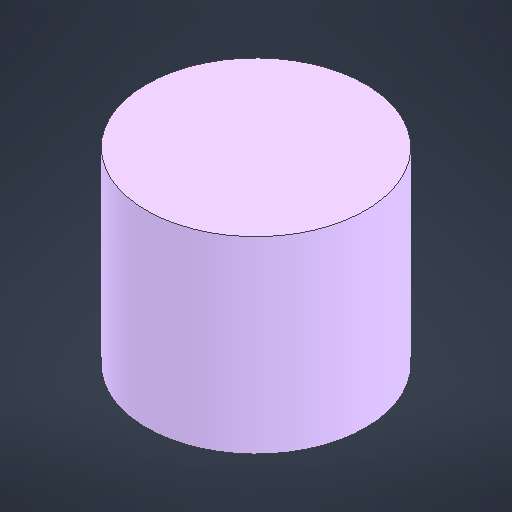
# Autodesk Inventor part: RotaryEncoderKnob
Saved by Autodesk Inventor 2026.2 (Build 302298000, 298)
## iProperties
Created: 2026-02-15
Part Number: RotaryEncoderKnob
Material: Generic
Document SubType Name: Modeling
Designer: bh
Density: 1 g/cm^3
Appearance: Default
Author: bh
Autodesk Inventor part; units mm, degrees
ref_plane "YZ Plane" through (0, 0, 0) normal (1, 0, 0) x (0, 1, 0)
ref_plane "XZ Plane" through (0, 0, 0) normal (0, 1, 0) x (-1, 0, 0)
ref_plane "XY Plane" through (0, 0, 0) normal (0, 0, 1) x (1, 0, 0)
sketch "Sketch2" plane through (0, 0, 0) normal (0, 1, 0) x (-1, 0, 0)
  circle A0 centre (0, 0) radius 10
  dimension "d0" = 20
  constraints: 1 centre point, 1 coincident
  measures "d0" diameter of A0
extrude "Extrusion1" add sketch "Sketch2" along normal blind 20
sketch "Sketch3" plane through (0, 0, 0) normal (0, -1, 0) x (1, 0, 0)
  circle A0 centre (0, 0) radius 4.15
  dimension "d3" = 8.3
  constraints: 1 centre point, 1 coincident
  measures "d3" diameter of A0
extrude "Extrusion2" cut sketch "Sketch3" against normal blind 12.4
sketch "Sketch4" plane through (0, 12.4, 0) normal (0, -1, 0) x (1, 0, 0)
  circle A0 centre (0, 0) radius 4.15 projected
  circle A1 centre (0, 0) radius 3.2
  line L0 (3.2, 0) -> (-1.7, 0)
  line L1 (-1.7, 0) -> (-1.7, -3.7858)
  line L2 (-1.7, 0) -> (-1.7, 3.7858)
  point P0 (-1.7, 2.7111)
  point P1 (-1.7, -2.7111)
  dimension "d16" = 6.4
  dimension "d17" = 4.9
  constraints: 6 end point, 2 point on circle, 1 coincident, 1 horizontal, 1 point on line, 1 vertical, 3 other
  measures "d17" distance of L0.start L0.end
extrude "Extrusion3" cut sketch "Sketch4" against normal blind 6.7 contours A1 L0 L2 | L1 L0 A1
sketch "Sketch8" plane through (0, 0, 0) normal (0, -1, 0) x (1, 0, 0)
  circle A0 centre (0, 0) radius 9.1
  dimension "d18" = 18.2
  constraints: 1 centre point, 1 coincident
  measures "d18" diameter of A0
extrude "Extrusion7" cut sketch "Sketch8" against normal blind 4.5
sketch "Sketch9" plane through (0, 0, 0) normal (0, -1, 0) x (1, 0, 0)
  circle A0 centre (0, 0) radius 10 projected
extrude "Extrusion8" cut sketch "Sketch9" against normal blind 2.8
sketch "Sketch10" plane through (0, 12.4, 0) normal (0, -1, 0) x (1, 0, 0)
  arc A0 (-1.7, -2.7111) -> (-1.7, 2.7111) centre (0, 0) ccw projected
  line L0 (-1.7, -2.7111) -> (-1.7, 2.7111) projected
  circle A1 centre (0, 0) radius 4.15 projected
extrude "Extrusion9" cut sketch "Sketch10" against normal blind 0.4
body "Solid1"
